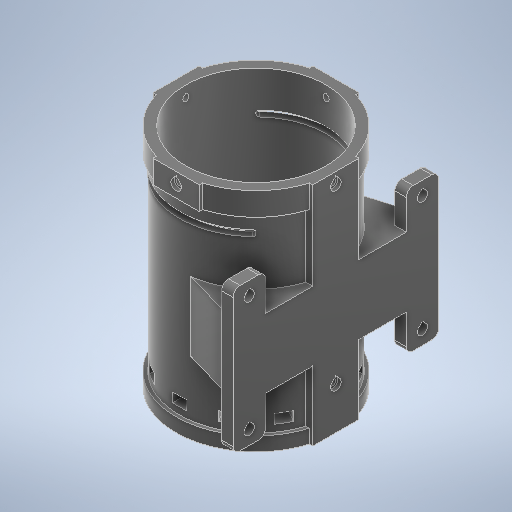
# Autodesk Inventor part: casing_cylindrical
Saved by Autodesk Inventor 2025 (Build 290162000, 162)
## iProperties
Created: 2026-08-03
Part Number: casing_cylindrical
Material: Ogólny
Document SubType Name: Modeling
Designer: zzapa
Density: 1 g/cm^3
Appearance: Gładki — czarny
Author: zzapa
Autodesk Inventor part; units mm, degrees
ref_plane "YZ Plane" through (0, 0, 0) normal (1, 0, 0) x (0, 1, 0)
ref_plane "XZ Plane" through (0, 0, 0) normal (0, 1, 0) x (-1, 0, 0)
sketch "Szkic1" plane through (0, 0, 0) normal (0, 0, 1) x (1, 0, 0)
  line L0 (-34.1596, 0) -> (44.6599, 0) projected
  line L1 (33.15, 90) -> (30.15, 90)
  line L2 (30.15, 90) -> (30.15, 0)
  line L3 (30.15, 0) -> (33.15, 0)
  line L4 (33.15, 0) -> (33.15, 90)
  line L5 (0, -27.6) -> (0, 109.6) projected
  line L6 (33.15, -8) -> (14.25, -8)
  line L7 (14.25, -8) -> (14.25, 0)
  line L8 (14.25, 0) -> (33.15, 0)
  line L9 (33.15, 0) -> (33.15, -8)
  line L10 (23, 6) -> (30.15, 6)
  line L11 (30.15, 6) -> (30.15, 0)
  line L12 (30.15, 0) -> (23, 0)
  line L13 (23, 0) -> (23, 6)
  point P0 (0, 0)
  point P1 (30.15, 0)
  point P2 (33.15, 0)
  point P3 (33.15, 0)
  point P4 (14.25, 0)
  point P5 (23, 0)
  dimension "d0" = 30.15
  dimension "d1" = 3
  dimension "d2" = 90
  dimension "d4" = 8
  dimension "d5" = 14.25
  dimension "d6" = 23
  dimension "d7" = 6
  constraints: 24 end point, 6 parallel, 5 collinear, 3 horizontal, 3 perpendicular
  measures "d0" distance from line of point (0, 0) L2
  measures "d1" distance of L1.start L1.end
  measures "d2" distance of L3.end L1.start
  measures "d4" distance of L6.end L7.end
  measures "d5" distance between parallel lines of L5 L7
  measures "d6" distance between parallel lines of L5 L13
  measures "d7" distance of L12.end L10.start
revolve "Obrót1" add sketch "Szkic1" angle 360 about axis through (0, -10, 0) along (0, 1, 0)
sketch "Szkic2" plane through (0, -8, 0) normal (0, -1, 0) x (1, 0, 0)
  circle A0 centre (0, 0) radius 33.15 projected
  line L0 (-34.6057, 10) -> (-31.6057, 10)
  line L1 (-31.6057, 10) -> (-31.6057, -10)
  line L2 (-31.6057, -10) -> (-34.6057, -10)
  line L3 (-34.6057, -10) -> (-34.6057, 10)
  line L4 (0, -46.76) -> (0, 46.76) projected
  line L5 (34.6057, 10) -> (31.6057, 10)
  line L6 (31.6057, 10) -> (31.6057, -10)
  line L7 (31.6057, -10) -> (34.6057, -10)
  line L8 (34.6057, -10) -> (34.6057, 10)
  line L9 (-48.815, 0) -> (48.815, 0) projected
  point P0 (-31.6057, 0)
  dimension "d10" = 20
  dimension "d11" = 3
  constraints: 16 end point, 4 symmetric about line, 2 parallel, 1 horizontal, 1 midpoint, 1 perpendicular, 1 point on line, 2 other
  measures "d10" distance of L2.end L0.start
  measures "d11" distance from line of L3 point (-31.606, 0)
extrude "Wyciągnięcie proste1" add sketch "Szkic2" against normal up to surface (98 mm away) contours L9 L6 A0 | L9 L8 L7 A0 | A0 L6 L9 | A0 L5 L8 L9 | L1 L9 A0 | A0 L9 L3 L0 | L2 L3 L9 A0 | A0 L9 L1
ref_plane "Płaszczyzna konstrukcyjna1" through (0, 41, 33.15) normal (0, 0, 1) x (1, 0, 0)
sketch "Szkic3" plane through (0, 41, 33.15) normal (0, 0, 1) x (1, 0, 0)
  line L0 (3, -40) -> (-3, -40)
  line L1 (-3, -40) -> (-3, -36)
  line L2 (-3, -36) -> (3, -36)
  line L3 (3, -36) -> (3, -40)
  line L4 (23, -41) -> (-23, -41) projected
  line L5 (23, -35) -> (-23, -35) projected
  line L6 (0, -35) -> (0, -41)
  line L7 (-3, -36) -> (3, -40)
  point P0 (0, -40)
  point P1 (0, -38)
  dimension "d17" = 4
  dimension "d18" = 6
  constraints: 12 end point, 4 midpoint, 2 parallel, 1 horizontal, 1 perpendicular
  measures "d17" distance of L2.end L0.start
  measures "d18" distance of L1.end L2.end
sketch "Szkic4" plane through (0, 6, 0) normal (0, 1, 0) x (1, 0, 0)
  arc A0 (-31.6057, -10) -> (31.6057, -10) centre (0, 0) ccw projected
  arc A1 (0, 0) -> (0, -33.15) centre (9999.9863, -16.575) ccw
  dimension "d19" = 10000
  constraints: 4 point on circle, 1 centre point, 1 coincident
  measures "d19" radius of A1
sweep "Przeciągnięcie1" cut profiles "Szkic3" path "Szkic4" path curves A1
pattern_circular "Szyk kołowy1" count 12 over 360 about axis through (0, -10, 0) along (0, 1, 0) of "Przeciągnięcie1" skipped copies 4 10
sketch "Szkic5" plane through (-34.6057, -8, 10) normal (0, -1, 0) x (1, 0, 0)
  line L0 (-13.8423, -10) -> (83.0538, -10) projected
  point P0 (34.6057, -10)
  point P1 (15.6057, -10)
  point P2 (44.1057, -26.4545)
  point P3 (44.1057, 6.4545)
  point P4 (34.6057, -10)
  dimension "d20" = 19
  dimension "d23" = 360
  constraints: 1 coincident, 1 point on line, 4 other
  measures "d20" distance of point (34.606, -10) point (15.606, -10)
hole "Otwór1" at (-19, -8, 0) at (9.5, -8, -16.4545) at (9.5, -8, 16.4545) direction (0, 1, 0) diameter 2.6 end through all
sketch "Szkic6" plane through (-34.6057, -8, -10) normal (-1, 0, 0) x (0, 0, 1)
  line L0 (10, -19.6) -> (10, 117.6) projected
  line L1 (20, 0) -> (0, 0) projected
  point P0 (10, 8)
  point P1 (10, 18.1)
  dimension "d35" = 18.1
  constraints: 1 point on line
  measures "d35" distance from line of L1 point (10, 18.1)
hole "Otwór2" at (-34.6057, 10.1, 0) direction (1, 0, 0) diameter 2.6 depth 34.6057 counterbore diameter 4.5 counterbore depth 1.5
mirror "Odbij1" about plane through (0, 0, 0) normal (1, 0, 0) of "Otwór2"
sketch "Szkic7" plane through (0, 0, 0) normal (1, 0, 0) x (0, 1, 0)
  line L0 (-27.6, 0) -> (109.6, 0) projected
  line L1 (74.3, 30.15) -> (71.7, 30.15)
  line L2 (71.7, 30.15) -> (71.7, 33.15)
  line L3 (71.7, 33.15) -> (74.3, 33.15)
  line L4 (74.3, 33.15) -> (74.3, 30.15)
  line L5 (5, 27.0908) -> (5, 30.0908) projected
  line L6 (5, 30.0908) -> (1, 30.0908) projected
  line L7 (1, 30.0908) -> (1, 27.0908) projected
  line L8 (1, 27.0908) -> (5, 27.0908) projected
  line L9 (5, 13.9087) -> (5, 19.1049) projected
  line L10 (5, 19.1049) -> (1, 19.1049) projected
  line L11 (1, 19.1049) -> (1, 13.9087) projected
  line L12 (1, 13.9087) -> (5, 13.9087) projected
  line L13 (1, 13.9091) -> (1, 19.1052) projected
  line L14 (1, 19.1052) -> (5, 19.1052) projected
  line L15 (5, 19.1052) -> (5, 13.9091) projected
  line L16 (5, 13.9091) -> (1, 13.9091) projected
  line L17 (1, 27.0911) -> (1, 30.091) projected
  line L18 (1, 30.091) -> (5, 30.091) projected
  line L19 (5, 30.091) -> (5, 27.0911) projected
  line L20 (5, 27.0911) -> (1, 27.0911) projected
  line L21 (1, 33.014) -> (1, 33.014) projected
  line L22 (1, 33.014) -> (5, 33.014) projected
  line L23 (5, 33.014) -> (5, 33.014) projected
  line L24 (5, 33.014) -> (1, 33.014) projected
  line L25 (-8, 10) -> (90, 10) projected
  line L26 (90, 10) -> (90, 10) projected
  line L27 (90, 10) -> (-8, 10) projected
  line L28 (-8, 10) -> (-8, 10) projected
  line L29 (-8, 33.15) -> (90, 33.15) projected
  line L30 (90, 30.15) -> (6, 30.15) projected
  line L31 (90, 10) -> (90, 33.15) projected
  point P0 (0, 0)
  point P1 (73, 30.15)
  dimension "d44" = 2.6
  dimension "d50" = 17
  constraints: 8 end point, 2 collinear, 2 parallel, 1 horizontal, 1 midpoint, 1 perpendicular
  measures "d44" distance of L2.end L3.end
  measures "d50" distance from line of point (73, 30.15) L31
revolve "Obrót2" cut sketch "Szkic7" angle 90 mid plane about axis through (0, -10, 0) along (0, 1, 0) contours L1 L2 L3 L4
fillet "Zaokrąglenie1" radius 1 4 edges at (-22.3799, 74.3, 22.3799) (-22.3799, 71.7, 22.3799) (22.3799, 74.3, 22.3799) (22.3799, 71.7, 22.3799)
mirror "Odbij2" about plane through (0, 0, 0) normal (0, 0, 1) of "Obrót2", "Zaokrąglenie1"
sketch "Szkic8" plane through (0, 41, 33.15) normal (0, 0, 1) x (1, 0, 0)
  line L0 (22.7228, 33.3) -> (-22.7228, 33.3) projected
  line L1 (-22.7228, 30.7) -> (22.7228, 30.7) projected
  line L2 (0, 33.3) -> (0, 30.7)
  point P0 (0, -41)
  point P1 (0, 30.7)
  point P2 (0, 32)
  point P3 (0, 32)
  constraints: 5 midpoint, 2 end point, 1 coincident, 1 vertical
sketch "Szkic12" plane through (0, 90, 0) normal (0, 1, 0) x (1, 0, 0)
  circle A0 centre (0, 0) radius 34.6057
  line L0 (-34.6057, -10) -> (-34.6057, 10) projected
  circle A1 centre (0, 0) radius 30.15
  circle A2 centre (0, 0) radius 30.15 projected
  point P0 (-34.6057, 0)
  constraints: 2 coincident, 1 centre point, 1 concentric, 1 horizontal alignment, 1 midpoint, 2 other
extrude "Wyciągnięcie proste5" add sketch "Szkic12" against normal blind 10
sketch "Szkic9" plane through (0, 0, 0) normal (0, 1, 0) x (1, 0, 0)
  circle A0 centre (0, 0) radius 23
  dimension "d51" = 46
  constraints: 1 centre point, 1 coincident
  measures "d51" diameter of A0
extrude "sleeve_cut" cut sketch "Szkic9" against normal blind 4
ref_plane "Płaszczyzna konstrukcyjna4" through (-34.6057, 22, 10) normal (0, -1, 0) x (1, 0, 0)
sketch "Szkic11" plane through (-34.6057, 22, 10) normal (0, -1, 0) x (1, 0, 0)
  arc A0 (3, -20) -> (66.2115, -20) centre (34.6057, -10) ccw projected
  line L0 (66.2115, -20) -> (69.2115, -20) projected
  line L1 (69.2115, -20) -> (69.2115, 0) projected
  circle A1 centre (34.6057, -10) radius 33.15
  line L2 (66.2115, -20) -> (69.2115, -20)
  line L3 (69.2115, -20) -> (69.2115, 0) projected
  line L4 (69.2115, -10) -> (69.2115, -50)
  line L5 (69.2115, -50) -> (64.2115, -50)
  line L6 (64.2115, -50) -> (39.2115, -42.8285)
  line L7 (-13.9471, -10) -> (83.6828, -10) projected
  line L8 (66.2115, 0) -> (69.2115, 0)
  line L9 (66.2115, 0) -> (69.2115, 0)
  line L10 (69.2115, -10) -> (69.2115, 30)
  line L11 (69.2115, 30) -> (64.2115, 30)
  line L12 (64.2115, 30) -> (64.2115, 30)
  line L13 (64.2115, 30) -> (39.2115, 22.8285)
  point P0 (39.2115, 22.8285)
  point P1 (66.2115, 0)
  point P2 (39.2115, -42.8285)
  dimension "d83" = 30
  dimension "d84" = 5
  dimension "d85" = 40
  constraints: 20 end point, 5 symmetric about line, 2 collinear, 1 coincident, 1 horizontal, 1 midpoint, 4 other
  measures "d83" distance from line of L4 L6.end
  measures "d84" distance of L4.end L5.end
  measures "d85" distance between parallel lines of L7 L5
extrude "Wyciągnięcie proste4" add sketch "Szkic11" against normal blind 30 contours A0 L0 L4 L5 L6 | L13 L11 L10 L8 A1
sketch "Szkic13" plane through (-34.6057, 90, 10) normal (0, 1, 0) x (1, 0, 0)
  arc A0 (1.4763, 0) -> (67.7351, 0) centre (34.6057, 10) ccw projected
  line L0 (34.6057, 58.815) -> (34.6057, -38.815) projected
  line L1 (24.6057, -24.6057) -> (44.6057, -24.6057)
  line L2 (44.6057, -24.6057) -> (44.6057, -21.6057)
  line L3 (44.6057, -21.6057) -> (24.6057, -21.6057)
  line L4 (24.6057, -21.6057) -> (24.6057, -24.6057)
  line L5 (-13.8423, 10) -> (83.0538, 10) projected
  line L6 (24.6057, 44.6057) -> (44.6057, 44.6057)
  line L7 (44.6057, 44.6057) -> (44.6057, 41.6057)
  line L8 (44.6057, 41.6057) -> (24.6057, 41.6057)
  line L9 (24.6057, 41.6057) -> (24.6057, 44.6057)
  point P0 (34.6057, -24.6057)
  point P1 (34.6057, 44.6057)
  dimension "d62" = 20
  dimension "d63" = 3
  constraints: 16 end point, 5 symmetric about line, 2 parallel, 1 horizontal, 1 midpoint, 1 perpendicular, 1 point on circle, 1 point on line
  measures "d62" distance of L1.start L1.end
  measures "d63" distance of L3.end L1.start
extrude "Wyciągnięcie proste6" add sketch "Szkic13" against normal up to surface (10 mm away)
sketch "Szkic14" plane through (10, 90, -34.6057) normal (0, 0, -1) x (-1, 0, 0)
  line L0 (0, 0) -> (20, 0) projected
  line L1 (20, -10) -> (0, -10) projected
  line L2 (10, 0) -> (10, -10)
  point P0 (10, -90)
  point P1 (10, -4.9)
  dimension "d76" = 4.9
  constraints: 2 end point, 2 midpoint, 1 point on line
  measures "d76" distance from line of point (10, -4.9) L0
hole "Otwór3" at (0, 85.1, -34.6057) direction (0, 0, 1) diameter 2.6 end up to face face through (0, 48, 0) facing (0, 1, 0) round with radius 30.15 far side no counterbore diameter 4.5 counterbore depth 1.5
pattern_circular "Szyk kołowy2" count 4 over 360 about axis through (0, -10, 0) along (0, 1, 0) of "Otwór3"
sketch "Szkic15" plane through (-34.6057, -8, 10) normal (0, -1, 0) x (1, 0, 0)
  arc A0 (1.4763, -20) -> (24.6057, -43.1294) centre (34.6057, -10) ccw projected
  arc A1 (3, -20) -> (66.2115, -20) centre (34.6057, -10) ccw projected
  circle A2 centre (34.6057, -10) radius 33.15
  circle A3 centre (34.6057, -10) radius 34.6057
  point P0 (24.6057, -43.1294)
  point P1 (1.4763, -20)
  point P2 (66.2115, -20)
  constraints: 2 centre point, 2 coincident, 2 concentric
extrude "Wyciągnięcie proste7" add sketch "Szkic15" against normal blind 6
sketch "Szkic16" plane through (34.6057, -8, 10) normal (1, 0, 0) x (0, 0, -1)
  line L0 (54.5, 14) -> (40.5, 14)
  line L1 (40.5, 14) -> (40.5, 76)
  line L2 (40.5, 76) -> (54.5, 76)
  line L3 (54.5, 76) -> (54.5, 14)
  line L4 (10, -19.6) -> (10, 117.6) projected
  line L5 (-34.5, 14) -> (-20.5, 14)
  line L6 (-20.5, 14) -> (-20.5, 76)
  line L7 (-20.5, 76) -> (-34.5, 76)
  line L8 (-34.5, 76) -> (-34.5, 14)
  line L9 (50, 30) -> (50, 60) projected
  line L10 (47.5, 14) -> (47.5, 76)
  line L11 (47.5, 20) -> (47.5, 70)
  line L12 (54.5, 45) -> (40.5, 45)
  point P0 (10, 8)
  point P1 (-27.5, 20)
  point P2 (-27.5, 70)
  point P3 (47.5, 45)
  point P4 (50, 45)
  dimension "d82" = 50
  dimension "d86" = 75
  dimension "d87" = 14
  dimension "d88" = 62
  dimension "d89" = 0
  constraints: 22 end point, 7 midpoint, 6 symmetric about line, 2 parallel, 1 horizontal, 1 perpendicular, 1 point on line
  measures "d82" distance of L11.end L11.start
  measures "d86" distance of point (-27.5, 20) L11.start
  measures "d87" distance of L0.start L0.end
  measures "d88" distance of L2.end L0.start
  measures "d89" horizontal distance of L11.start L11.end
extrude "Wyciągnięcie proste8" add sketch "Szkic16" against normal blind 5
sketch "Szkic17" plane through (29.6057, -8, 10) normal (-1, 0, 0) x (0, 0, 1)
  line L0 (-40.5, 14) -> (-40.5, 30) projected
  line L1 (-54.5, 76) -> (-54.5, 14) projected
  line L2 (-54.5, 14) -> (-40.5, 14) projected
  line L3 (-40.5, 76) -> (-54.5, 76) projected
  line L4 (-54.5, 45) -> (-40.5, 45)
  line L5 (-47.5, 76) -> (-47.5, 14)
  line L6 (-10, -19.6) -> (-10, 117.6) projected
  point P0 (-10, 8)
  point P1 (-47.5, 20)
  point P2 (-47.5, 70)
  point P3 (27.5, 20)
  point P4 (27.5, 70)
  dimension "d92" = 50
  constraints: 4 end point, 3 midpoint, 3 symmetric about line, 2 point on line, 1 horizontal
  measures "d92" distance of point (-47.5, 20) point (-47.5, 70)
hole "Otwór4" at (29.6057, 12, -37.5) at (29.6057, 62, -37.5) at (29.6057, 62, 37.5) at (29.6057, 12, 37.5) direction (1, 0, 0) diameter 4.3 end through all
fillet "Zaokrąglenie3" radius 3 8 edges at (32.1057, 68, -44.5) (32.1057, 6, -44.5) (32.1057, 6, -30.5) (32.1057, 6, 30.5) (32.1057, 6, 44.5) (32.1057, 68, 30.5) (32.1057, 68, 44.5) (32.1057, 68, -30.5)
sketch "Szkic18" plane through (29.6057, -8, 10) normal (-1, 0, 0) x (0, 0, 1)
  circle A0 centre (-47.5, 70) radius 2.15 projected
  line L0 (-47.5, 70) -> (-47.5, 74.3713)
  line L1 (-47.5, 73.0406) -> (-45.9797, 71.5203)
  line L2 (-47.5, 73.0406) -> (-49.0203, 71.5203)
  line L3 (-10, -19.6) -> (-10, 117.6) projected
  line L4 (-72.3, 8) -> (52.3, 8) projected
  circle A1 centre (-47.5, 70) radius 2.15
  line L5 (-47.5, 20) -> (-47.5, 24.3713)
  line L6 (-47.5, 23.0406) -> (-45.9797, 21.5203)
  line L7 (-47.5, 23.0406) -> (-49.0203, 21.5203)
  circle A2 centre (-47.5, 20) radius 2.15
  line L8 (27.5, 70) -> (27.5, 74.3713)
  line L9 (27.5, 73.0406) -> (29.0203, 71.5203)
  line L10 (27.5, 73.0406) -> (25.9797, 71.5203)
  circle A3 centre (27.5, 70) radius 2.15
  line L11 (27.5, 20) -> (27.5, 24.3713)
  line L12 (27.5, 23.0406) -> (29.0203, 21.5203)
  line L13 (27.5, 23.0406) -> (25.9797, 21.5203)
  circle A4 centre (27.5, 20) radius 2.15
  point P0 (-10, 8)
  dimension "d101" = 90
  dimension "d104" = 50
  dimension "d107" = 75
  constraints: 24 end point, 4 centre point, 4 coincident, 4 point on line, 2 vertical, 1 horizontal, 1 symmetric about line, 34 other
  measures "d101" angle of L1 L2
  measures "d104" distance of L0.start L5.start
  measures "d107" distance of L0.start L8.start
extrude "Wyciągnięcie proste9" cut sketch "Szkic18" against normal through all contours A0 L0 L1 | L2 L0 A0 | A2 L7 L5 | L5 L6 A2 | A3 L10 L8 | L8 L9 A3 | A4 L13 L11 | L11 L12 A4
sketch "Szkic19" plane through (34.6057, -8, 10) normal (1, 0, 0) x (0, 0, -1)
  circle A0 centre (10, 93.1) radius 2.25 projected
  circle A1 centre (10, 93.1) radius 2.25
  line L0 (10, 93.1) -> (10, 96.9784)
  line L1 (10, 96.282) -> (11.591, 94.691)
  line L2 (10, 96.282) -> (8.409, 94.691)
  point P0 (10, 18.1)
  dimension "d112" = 90
  constraints: 6 end point, 1 centre point, 1 coincident, 1 point on line, 1 symmetric about line, 1 vertical, 3 other
  measures "d112" angle of L1 L2
extrude "Wyciągnięcie proste10" cut sketch "Szkic19" against normal up to surface (1.5 mm away) contours A0 L0 L1 | L2 L0 A0
sketch "Szkic20" plane through (34.6057, -8, 10) normal (1, 0, 0) x (0, 0, -1)
  circle A0 centre (10, 93.1) radius 1.3 projected
  line L0 (10, 93.1) -> (10, 96.777)
  line L1 (10, 94.9385) -> (10.9192, 94.0192)
  line L2 (10, 94.9385) -> (9.0808, 94.0192)
  point P0 (10, 8)
  dimension "d116" = 90
  constraints: 6 end point, 1 midpoint, 1 symmetric about line, 1 vertical, 3 other
  measures "d116" angle of L2 L1
extrude "Wyciągnięcie proste11" cut sketch "Szkic20" against normal up to surface contours A0 L0 L1 | L2 L0 A0 round surface about axis through (0, 48, 0) along (0, 1, 0) radius 30.15 far side no
pattern_circular "Szyk kołowy3" count 4 over 360 about axis through (0, -10, 0) along (0, 1, 0) of "Wyciągnięcie proste11", "Wyciągnięcie proste10"
sketch "Szkic21" plane through (-34.6057, -8, -10) normal (-1, 0, 0) x (0, 0, 1)
  circle A0 centre (10, 18.1) radius 1.3 projected
  line L0 (10, 18.1) -> (10, 24.4715)
  line L1 (10.9192, 19.0192) -> (10, 19.9385)
  line L2 (9.0808, 19.0192) -> (10, 19.9385)
  point P0 (10, 8)
  dimension "d122" = 90
  constraints: 6 end point, 1 point on line, 1 symmetric about line, 1 vertical, 3 other
  measures "d122" angle of L1 L2
extrude "Wyciągnięcie proste12" cut sketch "Szkic21" against normal up to surface contours A0 L0 L1 | L2 L0 A0 round surface about axis through (0, 48, 0) along (0, 1, 0) radius 30.15 far side no
sketch "Szkic22" plane through (-34.6057, -8, -10) normal (-1, 0, 0) x (0, 0, 1)
  circle A0 centre (10, 18.1) radius 2.25 projected
  line L0 (10, 18.1) -> (10, 24.492)
  line L1 (10, 21.282) -> (11.591, 19.691)
  line L2 (10, 21.282) -> (8.409, 19.691)
  point P0 (10, 8)
  dimension "d125" = 90
  constraints: 6 end point, 1 point on line, 1 symmetric about line, 1 vertical, 3 other
  measures "d125" angle of L1 L2
extrude "Wyciągnięcie proste13" cut sketch "Szkic22" against normal up to surface (1.5 mm away) contours A0 L0 L1 | L2 L0 A0
pattern_circular "Szyk kołowy4" count 2 over 360 about axis through (0, -10, 0) along (0, 1, 0) of "Wyciągnięcie proste13", "Wyciągnięcie proste12"
sketch "Szkic23" plane through (34.6057, 90, 10) normal (0, 1, 0) x (1, 0, 0)
  circle A0 centre (-34.6057, 10) radius 30.35
  circle A1 centre (-34.6057, 10) radius 30.15
  circle A2 centre (-34.6057, 10) radius 30.15 projected
  dimension "d131" = 0.2
  constraints: 2 centre point, 2 coincident, 1 concentric
  measures "d131" radial gap between concentric circles of A0 A1
extrude "Wyciągnięcie proste14" cut sketch "Szkic23" against normal up to surface (84 mm away)
equation "\"d0\" = casing_r_in"
equation "\"d1\" = casing_d"
equation "\"d2\" = casing_h"
equation "\"d4\" = casing_lock_h"
equation "\"d5\" = casing_lock_hole_r"
equation "\"d6\" = casing_stator_fix_r"
equation "\"d7\" = casing_stator_fix_h"
equation "\"d10\" = casing_sidebar_width"
equation "\"d11\" = casing_sidebar_length"
equation "\"d17\" = casing_vent_hole_length"
equation "\"d18\" = casing_vent_hole_width"
equation "\"d19\" = casing_vent_hole_arc"
equation "\"d20\" = casing_head_insert_r"
equation "\"d25\" = insert_m2_pocket_d"
equation "\"d35\" = casing_radial_stator_insert_pos"
equation "\"d36\" = insert_m2_pocket_d"
equation "\"d38\" = insert_m2_pocket_D"
equation "\"d39\" = insert_m2_pocket_nut_h"
equation "\"d44\" = casing_cart_hole_width"
equation "\"d50\" = casing_cart_hole_pos"
equation "\"d43\" = casing_cart_hole_ang"
equation "\"d45\" = casing_cart_hole_corner"
equation "\"d51\" = casing_sleeve_cut_d"
equation "\"d52\" = casing_sleeve_cut_h"
equation "\"d83\" = casing_stand_cylinder_h"
equation "\"d84\" = casing_stand_foot_h"
equation "\"d85\" = casing_stand_foot_width"
equation "\"d57\" = casing_stand_width"
equation "\"d62\" = casing_sidebar_width"
equation "\"d63\" = casing_sidebar_length"
equation "\"d76\" = casing_backsleeve_insert_pos"
equation "\"d66\" = insert_m2_pocket_d"
equation "\"d68\" = insert_m2_pocket_D"
equation "\"d69\" = insert_m2_pocket_nut_h"
equation "\"d87\" = casing_stand_pad_a"
equation "\"d88\" = casing_stand_pad_b"
equation "\"stator_r_out\" = 30.15"
equation "\"stator_out_d\" = 3.2"
equation "\"stator_h\" = 45"
equation "\"mag_size_x\" = 7"
equation "\"mag_size_y\" = 3"
equation "\"mag_corner_r\" = 0.4"
equation "\"magnet_ring_r\" = 26.95"
equation "\"magnet_ring_d\" = 3.3"
equation "\"magnet_ring_h\" = 36"
equation "\"magnet_ring_pocket_mag_size_x\" = 7.1"
equation "\"magnet_ring_pocket_mag_size_y\" = 3.1"
equation "\"magnet_ring_pocket_mag_size_z\" = 10.1"
equation "\"magnet_ring_pocket_radial_cut\" = 1.4"
equation "\"casing_h\" = 90"
equation "\"casing_d\" = 3"
equation "\"casing_r_in\" = 30.15"
equation "\"rotor_core_r\" = 14.97"
equation "\"coil_groove_ang\" = 18"
equation "\"rotor_out_r\" = 22.5"
equation "\"rotor_coil_groove_in_r\" = 17"
equation "\"rotor_coil_groove_ang\" = 18deg"
equation "\"rotor_coil_groove_in_correction_r\" = 18"
equation "\"rotor_plastic_h\" = 32"
equation "\"rotor_teeth_d\" = 1.5"
equation "\"shaft_d\" = 8"
equation "\"insert25m_d\" = 2.9"
equation "\"insert25m_corner\" = 0.5"
equation "\"insert25m_h\" = 7"
equation "\"rotor_plastic_insert_r\" = 37"
equation "\"shaft_lock_1_d\" = 8.1"
equation "\"shaf_lock_1_D\" = 32"
equation "\"shaft_lock_1_D\" = 44"
equation "\"shaft_lock_1_h1\" = 3.5"
equation "\"shaft_lock_1_insert_part_h\" = 8"
equation "\"shaft_lock_1_corner\" = 2"
equation "\"shaft_lock_1_insert_part_a\" = 18"
equation "\"shaft_lock_2_h1\" = 3.5"
equation "\"shaft_lock_2_d\" = 8.1"
equation "\"shaft_lock_2_insert_part_a\" = 18"
equation "\"shaft_lock_2_D\" = 44"
equation "\"shaft_lock_2_corner\" = 2"
equation "\"shaft_lock_2_insert_part_h\" = 7"
equation "\"shaft_lock_2_rotor_insert_grove_d_in\" = 36"
equation "\"shaft_lock_2_rotor_insert_grove_width_out\" = 5.5"
equation "\"shaft_lock_2_rotor_insert_grove_width_in\" = 7.6"
equation "\"shaft_lock_2_rotor_insert_r\" = 37"
equation "\"shaft_lock_2_rotor_insert_screw_d\" = 2.6"
equation "\"insert25m_pocket_d\" = 2.6"
equation "\"insert25m_pocket_D\" = 4.5"
equation "\"insert25m_pocket_nut_h\" = 1.5"
equation "\"insert_m2_pocket_d\" = 2.6"
equation "\"insert_m2_h\" = 7"
equation "\"insert_m2_d\" = 2.9"
equation "\"insert_m2_corner\" = 0.5"
equation "\"insert_m2_pocket_D\" = 4.5"
equation "\"insert_m2_pocket_nut_h\" = 1.5"
equation "\"shaft_lock_1_insert_part_corner\" = 6"
equation "\"shaft_lock_1_insert_part_pos\" = 4"
equation "\"shaft_lock_1_rotor_insert_grove_width_in\" = 7.6"
equation "\"shaft_lock_1_rotor_insert_r\" = 37"
equation "\"shaft_lock_1_rotor_insert_grove_d_in\" = 36"
equation "\"shaft_lock_1_rotor_insert_grove_width_out\" = 5.5"
equation "\"shaft_lock_1_shaft_insert_axial_cut_out_width\" = 12"
equation "\"shaft_lock_1_shaft_insert_axial_cut_in_width\" = 5.4"
equation "\"shaft_lock_1_shaft_insert_corner\" = 2"
equation "\"shaft_lock_1_shaft_insert_corner_finish\" = 0.5"
equation "\"shaft_lock_1_shaft_insert_pos\" = 2.5"
equation "\"shaft_lock_2_shaft_insert_corner\" = 2"
equation "\"shaft_lock_2_shaft_insert_pos\" = 2.5"
equation "\"shaft_lock_2_shaft_insert_axial_cut_in_width\" = 5.4"
equation "\"shaft_lock_2_shaft_insert_axial_cut_out_width\" = 12"
equation "\"shaft_lock_2_shaft_insert_corner_finish\" = 0.5"
equation "\"commutator_plate_D\" = 22"
equation "\"commutator_plastic_d\" = 1"
equation "\"commutator_plastic_h\" = 17"
equation "\"commutator_plate_ang\" = 55deg"
equation "\"commutator_plate_d\" = 1"
equation "\"commutator_plate_h\" = 17"
equation "\"commutator_plastic_shaft_d\" = 8.1"
equation "\"commutator_plastic_insert_cut_deepness\" = 0.5"
equation "\"commutator_plastic_insert_cut_length\" = 6"
equation "\"commutator_plastic_insert_pos\" = 3"
equation "\"commutator_plate_insert_pos\" = 3"
equation "\"casing_lock_hole_r\" = 14.25"
equation "\"casing_lock_h\" = 8"
equation "\"casing_stator_fix_r\" = 23"
equation "\"casing_stator_fix_h\" = 6"
equation "\"magnet_ring_insert_part_lengthen\" = 8"
equation "\"casing_sidebar_width\" = 20"
equation "\"casing_sidebar_length\" = 3"
equation "\"casing_vent_hole_length\" = 4"
equation "\"casing_vent_hole_width\" = 6"
equation "\"casing_vent_hole_arc\" = 10000"
equation "\"sleeve_cup_r\" = 22"
equation "\"sleeve_cup_h\" = 4.5"
equation "\"sleeve_h\" = 7"
equation "\"sleeve_d\" = 3"
equation "\"sleeve_in_r\" = 11.1"
equation "\"casing_head_insert_r\" = 19"
equation "\"sleeve_head_insert_r\" = 19"
equation "\"magnet_ring_insert_part_radius_cut\" = 0.17"
equation "\"magnet_ring_insert_part_axial_flat_cut\" = 0.17"
equation "\"magnet_ring_insert_pos\" = 4"
equation "\"casing_radial_stator_insert_pos\" = 18.1"
equation "\"stator_radial_screw_d\" = 4"
equation "\"stator_radial_screw_pos\" = 4"
equation "\"rotor_sleeve_out_D\" = 10.5"
equation "\"rotor_sleeve_in_D\" = 8.15"
equation "\"rotor_sleeve_h\" = 32"
equation "\"carbon_brush_batt_h\" = 8"
equation "\"carbon_brush_batt_d\" = 4"
equation "\"brush_cart_outer_holder_width\" = 5.5"
equation "\"brush_cart_outer_holder_arc_r\" = 33.15"
equation "\"brush_cart_outer_holder_arc_pos\" = 1.5"
equation "\"casing_cart_hole_corner\" = 1"
equation "\"casing_cart_hole_width\" = 2.6"
equation "\"casing_cart_hole_ang\" = 90deg"
equation "\"brush_holder_batt_arc_r\" = 30.15"
equation "\"brush_holder_batt_width\" = 16"
equation "\"casing_sleeve_cut_d\" = 46"
equation "\"casing_sleeve_cut_h\" = 4"
equation "\"casing_stand_cylinder_h\" = 30"
equation "\"casing_stand_foot_h\" = 5"
equation "\"casing_stand_foot_width\" = 40"
equation "\"casing_stand_width\" = 30"
equation "\"casing_stand_pad_a\" = 14"
equation "\"casing_stand_pad_b\" = 62"
equation "\"casing_cart_hole_pos\" = 17"
equation "\"casing_backsleeve_insert_pos\" = 4.9"
